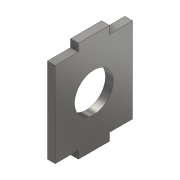
# Autodesk Inventor part: cover
Saved by Autodesk Inventor 2018.1 (Build 221171000, 171)
## iProperties
Created: 2019-06-27
Part Number: cover
Material: Сталь, углеродистая
Document SubType Name: ЛистМат
Designer: Boss
Mass: 6.17732 g
Surface Area: 10.3375 cm^2
Volume: 0.78692 cm^3
Density: 7.85 g/cm^3
Sheet Metal Rule: По умолчанию_мм
Appearance: С умеренной полировкой
Author: Boss
Autodesk Inventor part; units mm, degrees
ref_plane "YZ Plane" through (0, 0, 0) normal (1, 0, 0) x (0, 1, 0)
ref_plane "XZ Plane" through (0, 0, 0) normal (0, 1, 0) x (-1, 0, 0)
ref_plane "XY Plane" through (0, 0, 0) normal (0, 0, 1) x (1, 0, 0)
sketch "Эскиз1" plane through (0, 0, 0) normal (1, 0, 0) x (0, 1, 0)
  circle A0 centre (0, 0) radius 5
  line L0 (10, -11) -> (10, 11)
  line L1 (4, 13) -> (-4, 13)
  line L2 (-10, 11) -> (-10, -11)
  line L3 (4, 13) -> (4, 11)
  line L4 (4, 11) -> (10, 11)
  line L5 (0, 0) -> (0, 13.6398) construction
  line L6 (-4, 13) -> (-4, 11)
  line L7 (-4, 11) -> (-10, 11)
  line L8 (0, 0) -> (10.8227, 0) construction
  line L9 (4, -13) -> (-4, -13)
  line L10 (4, -13) -> (4, -11)
  line L11 (4, -11) -> (10, -11)
  line L12 (-4, -13) -> (-4, -11)
  line L13 (-4, -11) -> (-10, -11)
  dimension "d0" = 10
  dimension "d3" = 6
  dimension "d4" = 2
  dimension "d5" = 8
  dimension "d6" = 22
  measures "d0" diameter of A0
  measures "d3" distance of L0.end L3.end
  measures "d4" distance of L1.start L3.end
  measures "d5" distance of L1.start L1.end
  measures "d6" distance of L0.start L0.end
extrude "Пластина1" add sketch "Эскиз1" along normal blind 2
equation "\"d9\" = Толщина"
equation "\"Радиус_гибки\" = Толщина"
equation "\"Ширина_просечки\" = Толщина"
equation "\"Глубина_просечки\" = 0.5 * Толщина"
equation "\"Размер_просечки\" = 4 * Толщина"
equation "\"Мин_остаток\" = 2 * Толщина"
equation "\"Радиус_перехода\" = Радиус_гибки"
equation "\"Радиус_Якоби\" = Радиус_гибки"
equation "\"Размер_зазора\" = Толщина"
equation "\"Толщина\" = 2"
